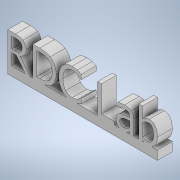
# Autodesk Inventor part: RDC_Lab
Saved by Autodesk Inventor 2021.4 (Build 254397000, 397)
## iProperties
Created: 2023-11-23
Part Number: RDC_Lab
Material: 一般
Document SubType Name: Modeling
Designer: ryusei
Density: 1 g/cm^3
Appearance: 既定
Author: ryusei
Autodesk Inventor part; units mm, degrees
ref_plane "YZ Plane" through (0, 0, 0) normal (1, 0, 0) x (0, 1, 0)
ref_plane "XZ Plane" through (0, 0, 0) normal (0, 1, 0) x (-1, 0, 0)
ref_plane "XY Plane" through (0, 0, 0) normal (0, 0, 1) x (1, 0, 0)
sketch "スケッチ1" plane through (0, 0, 0) normal (0, 0, 1) x (1, 0, 0)
  line L0 (-34.012, -0.0621) -> (23.7039, -0.0621) construction
  line L1 (23.7039, -0.0621) -> (23.7039, -12.2906) construction
  line L2 (23.7039, -12.2906) -> (-34.012, -12.2906) construction
  line L3 (-34.012, -12.2906) -> (-34.012, -0.0621) construction
  line L4 (-22.4393, -10.5078) -> (-24.1654, -10.5078)
  line L5 (-24.1654, -10.5078) -> (-27.3259, -6.5288)
  line L6 (-27.3259, -6.5288) -> (-28.8494, -6.5288)
  line L7 (-28.8494, -6.5288) -> (-28.8494, -10.5078)
  line L8 (-28.8494, -10.5078) -> (-30.1784, -10.5078)
  line L9 (-30.1784, -10.5078) -> (-30.1784, -0.5078)
  line L10 (-30.1784, -0.5078) -> (-27.6014, -0.5078)
  spline S0 degree 2 poles (-27.6014, -0.5078) (-26.7424, -0.5078) (-25.5836, -0.6941) (-25.0568, -1.0345) knots 0 0 0 1 2 2 2
  spline S1 degree 2 poles (-25.0568, -1.0345) (-24.5301, -1.3749) (-23.9223, -2.4364) (-23.9223, -3.2225) knots 0 0 0 1 2 2 2
  spline S2 degree 2 poles (-23.9223, -3.2225) (-23.9223, -4.3165) (-25.0406, -5.7995) (-25.9968, -6.1561) knots 0 0 0 1 2 2 2
  line L11 (-25.9968, -6.1561) -> (-22.4393, -10.5078)
  spline S3 degree 2 poles (-25.308, -3.3279) (-25.308, -2.8903) (-25.616, -2.2176) (-25.9401, -1.9988) knots 0 0 0 1 2 2 2
  spline S4 degree 2 poles (-25.9401, -1.9988) (-26.2237, -1.8125) (-26.9774, -1.6585) (-27.5284, -1.6585) knots 0 0 0 1 2 2 2
  line L12 (-27.5284, -1.6585) -> (-28.8494, -1.6585)
  line L13 (-28.8494, -1.6585) -> (-28.8494, -5.4186)
  line L14 (-28.8494, -5.4186) -> (-27.6824, -5.4186)
  spline S5 degree 2 poles (-27.6824, -5.4186) (-27.1071, -5.4186) (-26.1913, -5.216) (-25.8753, -4.9) knots 0 0 0 1 2 2 2
  spline S6 degree 2 poles (-25.8753, -4.9) (-25.5836, -4.6244) (-25.308, -3.8465) (-25.308, -3.3279) knots 0 0 0 1 2 2 2
  spline S7 degree 2 poles (-13.7602, -5.5159) (-13.7602, -6.8854) (-14.8704, -9.0896) (-15.8024, -9.7055) knots 0 0 0 1 2 2 2
  spline S8 degree 2 poles (-15.8024, -9.7055) (-16.5641, -10.1836) (-18.1281, -10.5078) (-19.3437, -10.5078) knots 0 0 0 1 2 2 2
  line L15 (-19.3437, -10.5078) -> (-21.6451, -10.5078)
  line L16 (-21.6451, -10.5078) -> (-21.6451, -0.5078)
  line L17 (-21.6451, -0.5078) -> (-19.368, -0.5078)
  spline S9 degree 2 poles (-19.368, -0.5078) (-17.9579, -0.5078) (-16.3534, -0.9292) (-15.7861, -1.3019) knots 0 0 0 1 2 2 2
  spline S10 degree 2 poles (-15.7861, -1.3019) (-14.8218, -1.9421) (-13.7602, -4.0572) (-13.7602, -5.5159) knots 0 0 0 1 2 2 2
  spline S11 degree 2 poles (-15.146, -5.4997) (-15.146, -4.3489) (-15.9077, -2.7201) (-16.6614, -2.2582) knots 0 0 0 1 2 2 2
  spline S12 degree 2 poles (-16.6614, -2.2582) (-17.1962, -1.9421) (-18.4037, -1.6585) (-19.3032, -1.6585) knots 0 0 0 1 2 2 2
  line L18 (-19.3032, -1.6585) -> (-20.3161, -1.6585)
  line L19 (-20.3161, -1.6585) -> (-20.3161, -9.357)
  line L20 (-20.3161, -9.357) -> (-19.3032, -9.357)
  spline S13 degree 2 poles (-19.3032, -9.357) (-18.4199, -9.357) (-17.0827, -9.0734) (-16.5398, -8.6925) knots 0 0 0 1 2 2 2
  spline S14 degree 2 poles (-16.5398, -8.6925) (-15.8429, -8.2225) (-15.146, -6.6666) (-15.146, -5.4997) knots 0 0 0 1 2 2 2
  spline S15 degree 2 poles (-8.4118, -10.686) (-9.3842, -10.686) (-11.0293, -10.0296) (-11.6289, -9.3732) knots 0 0 0 1 2 2 2
  spline S16 degree 2 poles (-11.6289, -9.3732) (-12.2286, -8.7249) (-12.885, -6.78) (-12.885, -5.5159) knots 0 0 0 1 2 2 2
  spline S17 degree 2 poles (-12.885, -5.5159) (-12.885, -4.2598) (-12.2448, -2.3959) (-11.637, -1.7071) knots 0 0 0 1 2 2 2
  spline S18 degree 2 poles (-11.637, -1.7071) (-11.0374, -1.0345) (-9.4004, -0.3295) (-8.3874, -0.3295) knots 0 0 0 1 2 2 2
  spline S19 degree 2 poles (-8.3874, -0.3295) (-7.885, -0.3295) (-7.0017, -0.4753) (-6.6289, -0.5888) knots 0 0 0 1 2 2 2
  spline S20 degree 2 poles (-6.6289, -0.5888) (-6.3048, -0.6941) (-5.6322, -0.994) (-5.2999, -1.1723) knots 0 0 0 1 2 2 2
  line L21 (-5.2999, -1.1723) -> (-5.2999, -2.7768)
  line L22 (-5.2999, -2.7768) -> (-5.4053, -2.7768)
  spline S21 degree 2 poles (-5.4053, -2.7768) (-5.5836, -2.6147) (-6.1346, -2.1609) (-6.5317, -1.9421) knots 0 0 0 1 2 2 2
  spline S22 degree 2 poles (-6.5317, -1.9421) (-6.9126, -1.7314) (-7.8121, -1.464) (-8.3955, -1.464) knots 0 0 0 1 2 2 2
  spline S23 degree 2 poles (-8.3955, -1.464) (-9.0357, -1.464) (-10.1784, -1.9907) (-10.6079, -2.4932) knots 0 0 0 1 2 2 2
  spline S24 degree 2 poles (-10.6079, -2.4932) (-11.0293, -3.0037) (-11.4993, -4.5515) (-11.4993, -5.5159) knots 0 0 0 1 2 2 2
  spline S25 degree 2 poles (-11.4993, -5.5159) (-11.4993, -6.545) (-11.0049, -8.028) (-10.5755, -8.5386) knots 0 0 0 1 2 2 2
  spline S26 degree 2 poles (-10.5755, -8.5386) (-10.1541, -9.0329) (-9.0276, -9.5353) (-8.3955, -9.5353) knots 0 0 0 1 2 2 2
  spline S27 degree 2 poles (-8.3955, -9.5353) (-7.8202, -9.5353) (-6.8396, -9.2517) (-6.4588, -9.041) knots 0 0 0 1 2 2 2
  spline S28 degree 2 poles (-6.4588, -9.041) (-6.0941, -8.8303) (-5.5511, -8.3927) (-5.3972, -8.2387) knots 0 0 0 1 2 2 2
  line L23 (-5.3972, -8.2387) -> (-5.2999, -8.2387)
  line L24 (-5.2999, -8.2387) -> (-5.2999, -9.827)
  spline S29 degree 2 poles (-5.2999, -9.827) (-5.6322, -9.981) (-6.2156, -10.2646) (-6.6289, -10.3943) knots 0 0 0 1 2 2 2
  spline S30 degree 2 poles (-6.6289, -10.3943) (-7.0665, -10.5402) (-7.8121, -10.686) (-8.4118, -10.686) knots 0 0 0 1 2 2 2
  line L25 (6.0291, -10.5078) -> (0.2349, -10.5078)
  line L26 (0.2349, -10.5078) -> (0.2349, -0.5078)
  line L27 (0.2349, -0.5078) -> (1.5639, -0.5078)
  line L28 (1.5639, -0.5078) -> (1.5639, -9.3246)
  line L29 (1.5639, -9.3246) -> (6.0291, -9.3246)
  line L30 (6.0291, -9.3246) -> (6.0291, -10.5078)
  spline S31 degree 2 poles (11.1587, -9.7136) (11.0048, -9.827) (10.4861, -10.2322) (10.243, -10.3538) knots 0 0 0 1 2 2 2
  spline S32 degree 2 poles (10.243, -10.3538) (9.9108, -10.5321) (9.2868, -10.7185) (8.7195, -10.7185) knots 0 0 0 1 2 2 2
  spline S33 degree 2 poles (8.7195, -10.7185) (8.2576, -10.7185) (7.4229, -10.37) (7.1069, -10.0539) knots 0 0 0 1 2 2 2
  spline S34 degree 2 poles (7.1069, -10.0539) (6.807, -9.746) (6.4424, -8.8384) (6.4424, -8.336) knots 0 0 0 1 2 2 2
  spline S35 degree 2 poles (6.4424, -8.336) (6.4424, -7.558) (7.0988, -6.4559) (7.8119, -6.1398) knots 0 0 0 1 2 2 2
  spline S36 degree 2 poles (7.8119, -6.1398) (8.444, -5.8481) (10.162, -5.6293) (11.1587, -5.5726) knots 0 0 0 1 2 2 2
  line L31 (11.1587, -5.5726) -> (11.1587, -5.3295)
  spline S37 degree 2 poles (11.1587, -5.3295) (11.1587, -4.8919) (10.8913, -4.3489) (10.6482, -4.195) knots 0 0 0 1 2 2 2
  spline S38 degree 2 poles (10.6482, -4.195) (10.4051, -4.041) (9.7082, -3.9437) (9.3354, -3.9437) knots 0 0 0 1 2 2 2
  spline S39 degree 2 poles (9.3354, -3.9437) (8.8978, -3.9437) (7.7147, -4.2031) (7.1231, -4.4543) knots 0 0 0 1 2 2 2
  line L32 (7.1231, -4.4543) -> (7.0502, -4.4543)
  line L33 (7.0502, -4.4543) -> (7.0502, -3.1658)
  spline S40 degree 2 poles (7.0502, -3.1658) (7.3986, -3.0685) (8.7033, -2.8254) (9.3435, -2.8254) knots 0 0 0 1 2 2 2
  spline S41 degree 2 poles (9.3435, -2.8254) (10.1215, -2.8254) (11.1831, -3.0685) (11.6045, -3.3846) knots 0 0 0 1 2 2 2
  spline S42 degree 2 poles (11.6045, -3.3846) (12.0177, -3.6925) (12.4229, -4.6731) (12.4229, -5.3781) knots 0 0 0 1 2 2 2
  line L34 (12.4229, -5.3781) -> (12.4229, -10.5078)
  line L35 (12.4229, -10.5078) -> (11.1587, -10.5078)
  line L36 (11.1587, -10.5078) -> (11.1587, -9.7136)
  line L37 (11.1587, -8.6601) -> (11.1587, -6.5774)
  spline S43 degree 2 poles (11.1587, -6.5774) (10.7049, -6.618) (9.3354, -6.7557) (8.9059, -6.8854) knots 0 0 0 1 2 2 2
  spline S44 degree 2 poles (8.9059, -6.8854) (8.4035, -7.0394) (7.7471, -7.6796) (7.7471, -8.2468) knots 0 0 0 1 2 2 2
  spline S45 degree 2 poles (7.7471, -8.2468) (7.7471, -8.8951) (8.4764, -9.5515) (9.1733, -9.5515) knots 0 0 0 1 2 2 2
  spline S46 degree 2 poles (9.1733, -9.5515) (9.7649, -9.5515) (10.7374, -9.041) (11.1587, -8.6601) knots 0 0 0 1 2 2 2
  spline S47 degree 2 poles (20.4861, -6.6342) (20.4861, -8.4737) (18.7033, -10.7185) (17.3581, -10.7185) knots 0 0 0 1 2 2 2
  spline S48 degree 2 poles (17.3581, -10.7185) (16.7503, -10.7185) (15.8832, -10.4186) (15.4618, -10.1593) knots 0 0 0 1 2 2 2
  line L38 (15.4618, -10.1593) -> (15.3808, -10.5078)
  line L39 (15.3808, -10.5078) -> (14.1976, -10.5078)
  line L40 (14.1976, -10.5078) -> (14.1976, -0.0621)
  line L41 (14.1976, -0.0621) -> (15.4618, -0.0621)
  line L42 (15.4618, -0.0621) -> (15.4618, -3.7898)
  spline S49 degree 2 poles (15.4618, -3.7898) (15.9399, -3.3603) (17.0502, -2.793) (17.7552, -2.793) knots 0 0 0 1 2 2 2
  spline S50 degree 2 poles (17.7552, -2.793) (19.0275, -2.793) (20.4861, -4.827) (20.4861, -6.6342) knots 0 0 0 1 2 2 2
  spline S51 degree 2 poles (19.1814, -6.7314) (19.1814, -5.3862) (18.363, -3.9924) (17.4553, -3.9924) knots 0 0 0 1 2 2 2
  spline S52 degree 2 poles (17.4553, -3.9924) (16.9448, -3.9924) (15.8913, -4.4786) (15.4618, -4.8514) knots 0 0 0 1 2 2 2
  line L43 (15.4618, -4.8514) -> (15.4618, -9.1544)
  spline S53 degree 2 poles (15.4618, -9.1544) (15.9399, -9.3894) (16.6774, -9.5839) (17.115, -9.5839) knots 0 0 0 1 2 2 2
  spline S54 degree 2 poles (17.115, -9.5839) (18.0793, -9.5839) (19.1814, -8.2144) (19.1814, -6.7314) knots 0 0 0 1 2 2 2
  point P0 (0, 0)
  constraints: 2 other
extrude "押し出し1" add sketch "スケッチ1" along normal blind 5
sketch "スケッチ2" plane through (0.2349, -10.5078, 0) normal (0, -1, 0) x (1, 0, 0)
  line L0 (-30.4133, 0) -> (-30.4133, 5) projected
  line L1 (20.2512, 0) -> (20.2512, 5) projected
  line L2 (-30.4133, 5) -> (20.2512, 5)
  line L3 (20.2512, 5) -> (20.2512, 0)
  line L4 (20.2512, 0) -> (-30.4133, 0)
  line L5 (-30.4133, 0) -> (-30.4133, 5)
  point P0 (-0.2349, 0)
  constraints: 8 end point, 2 parallel, 1 horizontal, 1 perpendicular
extrude "押し出し2" add sketch "スケッチ2" along normal blind 3 and the other way blind 0.1
